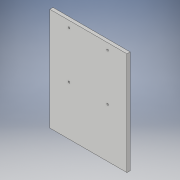
# Autodesk Inventor part: Robot_Base
Saved by Autodesk Inventor 2019.4 (Build 234330000, 330)
## iProperties
Created: 2019-09-20
Part Number: Robot_Base
Material: Generic
Document SubType Name: Modeling
Designer: Pranav Maddula
Density: 1 g/cm^3
Appearance: Default
Author: Pranav Maddula
Autodesk Inventor part; units mm, degrees
ref_plane "YZ Plane" through (0, 0, 0) normal (1, 0, 0) x (0, 1, 0)
ref_plane "XZ Plane" through (0, 0, 0) normal (0, 1, 0) x (-1, 0, 0)
ref_plane "XY Plane" through (0, 0, 0) normal (0, 0, 1) x (1, 0, 0)
sketch "Sketch1" plane through (0, 0, 0) normal (0, 0, 1) x (1, 0, 0)
  line L0 (-57.3998, 94.2737) -> (95.0002, 94.2737)
  line L1 (95.0002, 94.2737) -> (95.0002, -108.9263)
  line L2 (95.0002, -108.9263) -> (-57.3998, -108.9263)
  line L3 (-57.3998, -108.9263) -> (-57.3998, 94.2737)
  point P0 (0, 0)
  dimension "d0" = 152.4
  dimension "d1" = 203.2
  constraints: 8 end point, 2 parallel, 1 horizontal, 1 perpendicular
  measures "d0" distance of L0.start L0.end
  measures "d1" distance of L0.end L1.end
extrude "Extrusion1" add sketch "Sketch1" along normal blind 6.35
sketch "Sketch3" plane through (0, 0, 6.35) normal (0, 0, 1) x (1, 0, 0)
  circle A0 centre (-19.2998, 81.5737) radius 1.7145
  line L0 (-57.3998, 94.2737) -> (-57.3998, -108.9263) projected
  circle A1 centre (56.9002, 81.5737) radius 1.7145
  circle A2 centre (-19.2998, -11.1363) radius 1.7145
  circle A3 centre (56.9002, -11.1363) radius 1.7145
  line L1 (95.0002, -108.9263) -> (95.0002, 94.2737) projected
  line L2 (95.0002, 94.2737) -> (-57.3998, 94.2737) projected
  point P0 (0, 0)
  dimension "d4" = 3.429
  dimension "d7" = 38.1
  dimension "d14" = 3.429
  dimension "d15" = 3.429
  dimension "d16" = 3.429
  dimension "d17" = 76.2
  dimension "d18" = 92.71
  dimension "d19" = 92.71
  dimension "d20" = 76.2
  dimension "d21" = 38.1
  dimension "d22" = 12.7
  dimension "d23" = 12.7
  constraints: 4 centre point
  measures "d4" diameter of A0
  measures "d7" distance from line of L0 A0.centre
  measures "d14" diameter of A1
  measures "d15" diameter of A2
  measures "d16" diameter of A3
  measures "d17" distance of A1.centre A0.centre
  measures "d18" distance of A2.centre A0.centre
  measures "d19" distance of A3.centre A1.centre
  measures "d20" distance of A3.centre A2.centre
  measures "d21" distance from line of L1 A3.centre
  measures "d22" distance from line of L2 A0.centre
  measures "d23" distance from line of L2 A1.centre
extrude "Extrusion2" cut sketch "Sketch3" against normal blind 6.35
body "Solid1"
